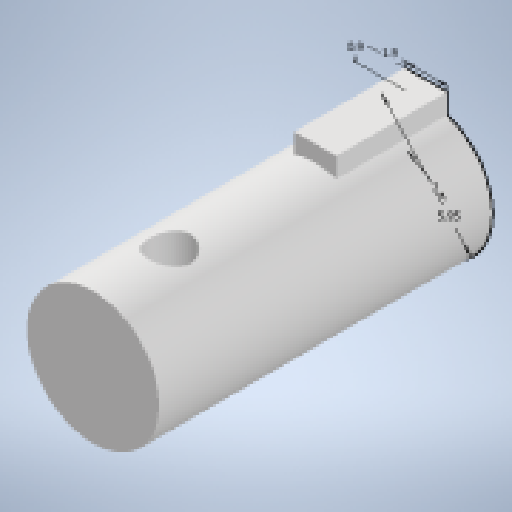
# Autodesk Inventor part: NAN_tower_mount_mk2
Saved by Autodesk Inventor 2024 (Build 280153000, 153)
## iProperties
Created: 2023-06-22
Part Number: NAN_tower_mount_mk2
Material: Generic
Document SubType Name: Modeling
Designer: Rober
Density: 1 g/cm^3
Appearance: Default
Author: Rober
Autodesk Inventor part; units mm, degrees
ref_plane "YZ Plane" through (0, 0, 0) normal (1, 0, 0) x (0, 1, 0)
ref_plane "XZ Plane" through (0, 0, 0) normal (0, 1, 0) x (-1, 0, 0)
sketch "Sketch3" plane through (0, 0, 0) normal (0, 0, 1) x (1, 0, 0)
  circle A0 centre (0, 0) radius 2.975
  line L0 (-0.95, 3.7192) -> (0.95, 3.7192)
  line L1 (0.95, 3.7192) -> (0.95, 2.8192)
  line L2 (-0.95, 2.8192) -> (-0.95, 3.7192)
  circle A1 centre (0, 0) radius 1
  dimension "d6" = 5.95
  dimension "d9" = 1.9
  dimension "d10" = 0.9
  dimension "d11" = 2
  constraints: 6 end point, 2 centre point, 2 coincident, 2 parallel, 2 point on circle, 1 horizontal, 1 perpendicular
  measures "d6" diameter of A0
  measures "d9" distance of L0.start L0.end
  measures "d10" distance of L2.start L0.start
  measures "d11" diameter of A1
extrude "Extrusion1" add sketch "Sketch3" along normal blind 15 contours A0 | A1
extrude "Extrusion2" add sketch "Sketch3" along normal blind 5 fills toward (-0.9, 3.2692) open curves L2 L0 L1
extrude "Extrusion3" cut sketch "Sketch3" along normal blind 10 contours A1
ref_plane "Work Plane1" through (0, 2.975, 0) normal (0, 1, 0) x (1, 0, 0)
sketch "Sketch4" plane through (0, 2.975, 0) normal (0, 1, 0) x (1, 0, 0)
  circle A0 centre (0, -11.55) radius 0.95
  line L0 (-2.975, -15) -> (2.975, -15) projected
  point P0 (0, 0)
  dimension "d17" = 1.9
  dimension "d18" = 3.45
  constraints: 1 centre point
  measures "d17" diameter of A0
  measures "d18" distance from line of L0 A0.centre
extrude "Extrusion4" cut sketch "Sketch4" against normal through all
body "Solid2"
